Autodesk Inventor part; units mm, degrees
(part 5 of 15)
  line L847 (11.116, -14.792) -> (11.116, -15.808)
  arc A1970 (11.0652, -15.808) -> (11.1668, -15.808) centre (11.116, -15.808) ccw
  arc A1971 (11.1668, -14.792) -> (11.0652, -14.792) centre (11.116, -14.792) ccw
  arc A1972 (66.7332, 38.092) -> (66.8348, 38.092) centre (66.784, 38.092) ccw
  line L848 (7.084, -14.792) -> (9.116, -14.792)
  arc A1973 (9.116, -14.8428) -> (9.116, -14.7412) centre (9.116, -14.792) ccw
  arc A1974 (7.084, -14.7412) -> (7.084, -14.8428) centre (7.084, -14.792) ccw
  line L849 (9.116, -14.792) -> (9.116, -15.808)
  arc A1975 (9.0652, -15.808) -> (9.1668, -15.808) centre (9.116, -15.808) ccw
  arc A1976 (9.1668, -14.792) -> (9.0652, -14.792) centre (9.116, -14.792) ccw
  line L850 (9.116, -15.808) -> (7.084, -15.808)
  arc A1977 (7.084, -15.7572) -> (7.084, -15.8588) centre (7.084, -15.808) ccw
  arc A1978 (9.116, -15.8588) -> (9.116, -15.7572) centre (9.116, -15.808) ccw
  line L851 (7.084, -15.808) -> (7.084, -14.792)
  arc A1979 (7.1348, -14.792) -> (7.0332, -14.792) centre (7.084, -14.792) ccw
  arc A1980 (7.0332, -15.808) -> (7.1348, -15.808) centre (7.084, -15.808) ccw
  line L852 (5.316, 47.992) -> (3.284, 47.992)
  line L853 (11.116, -23.808) -> (9.084, -23.808)
  arc A1981 (9.084, -23.7572) -> (9.084, -23.8588) centre (9.084, -23.808) ccw
  arc A1982 (11.116, -23.8588) -> (11.116, -23.7572) centre (11.116, -23.808) ccw
  line L854 (9.084, -23.808) -> (9.084, -22.792)
  arc A1983 (9.1348, -22.792) -> (9.0332, -22.792) centre (9.084, -22.792) ccw
  arc A1984 (9.0332, -23.808) -> (9.1348, -23.808) centre (9.084, -23.808) ccw
  line L855 (9.084, -22.792) -> (11.116, -22.792)
  arc A1985 (11.116, -22.8428) -> (11.116, -22.7412) centre (11.116, -22.792) ccw
  arc A1986 (9.084, -22.7412) -> (9.084, -22.8428) centre (9.084, -22.792) ccw
  line L856 (11.116, -22.792) -> (11.116, -23.808)
  arc A1987 (11.0652, -23.808) -> (11.1668, -23.808) centre (11.116, -23.808) ccw
  arc A1988 (11.1668, -22.792) -> (11.0652, -22.792) centre (11.116, -22.792) ccw
  arc A1989 (3.284, 48.0428) -> (3.284, 47.9412) centre (3.284, 47.992) ccw
  line L857 (9.116, -23.808) -> (7.084, -23.808)
  arc A1990 (7.084, -23.7572) -> (7.084, -23.8588) centre (7.084, -23.808) ccw
  arc A1991 (9.116, -23.8588) -> (9.116, -23.7572) centre (9.116, -23.808) ccw
  line L858 (7.084, -23.808) -> (7.084, -22.792)
  arc A1992 (7.1348, -22.792) -> (7.0332, -22.792) centre (7.084, -22.792) ccw
  arc A1993 (7.0332, -23.808) -> (7.1348, -23.808) centre (7.084, -23.808) ccw
  line L859 (7.084, -22.792) -> (9.116, -22.792)
  arc A1994 (9.116, -22.8428) -> (9.116, -22.7412) centre (9.116, -22.792) ccw
  arc A1995 (7.084, -22.7412) -> (7.084, -22.8428) centre (7.084, -22.792) ccw
  line L860 (9.116, -22.792) -> (9.116, -23.808)
  arc A1996 (9.0652, -23.808) -> (9.1668, -23.808) centre (9.116, -23.808) ccw
  arc A1997 (9.1668, -22.792) -> (9.0652, -22.792) centre (9.116, -22.792) ccw
  arc A1998 (5.316, 47.9412) -> (5.316, 48.0428) centre (5.316, 47.992) ccw
  line L861 (8.884, -18.292) -> (10.916, -18.292)
  arc A1999 (10.916, -18.3428) -> (10.916, -18.2412) centre (10.916, -18.292) ccw
  arc A2000 (8.884, -18.2412) -> (8.884, -18.3428) centre (8.884, -18.292) ccw
  line L862 (10.916, -18.292) -> (10.916, -19.308)
  arc A2001 (10.8652, -19.308) -> (10.9668, -19.308) centre (10.916, -19.308) ccw
  arc A2002 (10.9668, -18.292) -> (10.8652, -18.292) centre (10.916, -18.292) ccw
  line L863 (10.916, -19.308) -> (8.884, -19.308)
  arc A2003 (8.884, -19.2572) -> (8.884, -19.3588) centre (8.884, -19.308) ccw
  arc A2004 (10.916, -19.3588) -> (10.916, -19.2572) centre (10.916, -19.308) ccw
  line L864 (8.884, -19.308) -> (8.884, -18.292)
  arc A2005 (8.9348, -18.292) -> (8.8332, -18.292) centre (8.884, -18.292) ccw
  arc A2006 (8.8332, -19.308) -> (8.9348, -19.308) centre (8.884, -19.308) ccw
  line L865 (3.284, 47.992) -> (3.284, 49.008)
  line L866 (0.916, -15.808) -> (-1.116, -15.808)
  arc A2007 (-1.116, -15.7572) -> (-1.116, -15.8588) centre (-1.116, -15.808) ccw
  arc A2008 (0.916, -15.8588) -> (0.916, -15.7572) centre (0.916, -15.808) ccw
  line L867 (-1.116, -15.808) -> (-1.116, -14.792)
  arc A2009 (-1.0652, -14.792) -> (-1.1668, -14.792) centre (-1.116, -14.792) ccw
  arc A2010 (-1.1668, -15.808) -> (-1.0652, -15.808) centre (-1.116, -15.808) ccw
  line L868 (-1.116, -14.792) -> (0.916, -14.792)
  arc A2011 (0.916, -14.8428) -> (0.916, -14.7412) centre (0.916, -14.792) ccw
  arc A2012 (-1.116, -14.7412) -> (-1.116, -14.8428) centre (-1.116, -14.792) ccw
  line L869 (0.916, -14.792) -> (0.916, -15.808)
  arc A2013 (0.8652, -15.808) -> (0.9668, -15.808) centre (0.916, -15.808) ccw
  arc A2014 (0.9668, -14.792) -> (0.8652, -14.792) centre (0.916, -14.792) ccw
  arc A2015 (3.3348, 49.008) -> (3.2332, 49.008) centre (3.284, 49.008) ccw
  line L870 (4.916, -15.808) -> (2.884, -15.808)
  arc A2016 (2.884, -15.7572) -> (2.884, -15.8588) centre (2.884, -15.808) ccw
  arc A2017 (4.916, -15.8588) -> (4.916, -15.7572) centre (4.916, -15.808) ccw
  line L871 (2.884, -15.808) -> (2.884, -14.792)
  arc A2018 (2.9348, -14.792) -> (2.8332, -14.792) centre (2.884, -14.792) ccw
  arc A2019 (2.8332, -15.808) -> (2.9348, -15.808) centre (2.884, -15.808) ccw
  line L872 (2.884, -14.792) -> (4.916, -14.792)
  arc A2020 (4.916, -14.8428) -> (4.916, -14.7412) centre (4.916, -14.792) ccw
  arc A2021 (2.884, -14.7412) -> (2.884, -14.8428) centre (2.884, -14.792) ccw
  line L873 (4.916, -14.792) -> (4.916, -15.808)
  arc A2022 (4.8652, -15.808) -> (4.9668, -15.808) centre (4.916, -15.808) ccw
  arc A2023 (4.9668, -14.792) -> (4.8652, -14.792) centre (4.916, -14.792) ccw
  arc A2024 (3.2332, 47.992) -> (3.3348, 47.992) centre (3.284, 47.992) ccw
  line L874 (8.884, -19.292) -> (10.916, -19.292)
  arc A2025 (10.916, -19.3428) -> (10.916, -19.2412) centre (10.916, -19.292) ccw
  arc A2026 (8.884, -19.2412) -> (8.884, -19.3428) centre (8.884, -19.292) ccw
  line L875 (10.916, -19.292) -> (10.916, -20.308)
  arc A2027 (10.8652, -20.308) -> (10.9668, -20.308) centre (10.916, -20.308) ccw
  arc A2028 (10.9668, -19.292) -> (10.8652, -19.292) centre (10.916, -19.292) ccw
  line L876 (10.916, -20.308) -> (8.884, -20.308)
  arc A2029 (8.884, -20.2572) -> (8.884, -20.3588) centre (8.884, -20.308) ccw
  arc A2030 (10.916, -20.3588) -> (10.916, -20.2572) centre (10.916, -20.308) ccw
  line L877 (8.884, -20.308) -> (8.884, -19.292)
  arc A2031 (8.9348, -19.292) -> (8.8332, -19.292) centre (8.884, -19.292) ccw
  arc A2032 (8.8332, -20.308) -> (8.9348, -20.308) centre (8.884, -20.308) ccw
  line L878 (3.284, 49.008) -> (5.316, 49.008)
  line L879 (2.916, -23.808) -> (0.884, -23.808)
  arc A2033 (0.884, -23.7572) -> (0.884, -23.8588) centre (0.884, -23.808) ccw
  arc A2034 (2.916, -23.8588) -> (2.916, -23.7572) centre (2.916, -23.808) ccw
  line L880 (0.884, -23.808) -> (0.884, -22.792)
  arc A2035 (0.9348, -22.792) -> (0.8332, -22.792) centre (0.884, -22.792) ccw
  arc A2036 (0.8332, -23.808) -> (0.9348, -23.808) centre (0.884, -23.808) ccw
  line L881 (0.884, -22.792) -> (2.916, -22.792)
  arc A2037 (2.916, -22.8428) -> (2.916, -22.7412) centre (2.916, -22.792) ccw
  arc A2038 (0.884, -22.7412) -> (0.884, -22.8428) centre (0.884, -22.792) ccw
  line L882 (2.916, -22.792) -> (2.916, -23.808)
  arc A2039 (2.8652, -23.808) -> (2.9668, -23.808) centre (2.916, -23.808) ccw
  arc A2040 (2.9668, -22.792) -> (2.8652, -22.792) centre (2.916, -22.792) ccw
  arc A2041 (5.316, 48.9572) -> (5.316, 49.0588) centre (5.316, 49.008) ccw
  line L883 (0.916, -23.808) -> (-1.116, -23.808)
  arc A2042 (-1.116, -23.7572) -> (-1.116, -23.8588) centre (-1.116, -23.808) ccw
  arc A2043 (0.916, -23.8588) -> (0.916, -23.7572) centre (0.916, -23.808) ccw
  line L884 (-1.116, -23.808) -> (-1.116, -22.792)
  arc A2044 (-1.0652, -22.792) -> (-1.1668, -22.792) centre (-1.116, -22.792) ccw
  arc A2045 (-1.1668, -23.808) -> (-1.0652, -23.808) centre (-1.116, -23.808) ccw
  line L885 (-1.116, -22.792) -> (0.916, -22.792)
  arc A2046 (0.916, -22.8428) -> (0.916, -22.7412) centre (0.916, -22.792) ccw
  arc A2047 (-1.116, -22.7412) -> (-1.116, -22.8428) centre (-1.116, -22.792) ccw
  line L886 (0.916, -22.792) -> (0.916, -23.808)
  arc A2048 (0.8652, -23.808) -> (0.9668, -23.808) centre (0.916, -23.808) ccw
  arc A2049 (0.9668, -22.792) -> (0.8652, -22.792) centre (0.916, -22.792) ccw
  arc A2050 (3.284, 49.0588) -> (3.284, 48.9572) centre (3.284, 49.008) ccw
  line L887 (3.716, -19.808) -> (1.684, -19.808)
  arc A2051 (1.684, -19.7572) -> (1.684, -19.8588) centre (1.684, -19.808) ccw
  arc A2052 (3.716, -19.8588) -> (3.716, -19.7572) centre (3.716, -19.808) ccw
  line L888 (1.684, -19.808) -> (1.684, -18.792)
  arc A2053 (1.7348, -18.792) -> (1.6332, -18.792) centre (1.684, -18.792) ccw
  arc A2054 (1.6332, -19.808) -> (1.7348, -19.808) centre (1.684, -19.808) ccw
  line L889 (1.684, -18.792) -> (3.716, -18.792)
  arc A2055 (3.716, -18.8428) -> (3.716, -18.7412) centre (3.716, -18.792) ccw
  arc A2056 (1.684, -18.7412) -> (1.684, -18.8428) centre (1.684, -18.792) ccw
  line L890 (3.716, -18.792) -> (3.716, -19.808)
  arc A2057 (3.6652, -19.808) -> (3.7668, -19.808) centre (3.716, -19.808) ccw
  arc A2058 (3.7668, -18.792) -> (3.6652, -18.792) centre (3.716, -18.792) ccw
  line L891 (5.316, 49.008) -> (5.316, 47.992)
  line L892 (-11.108, -24.116) -> (-11.108, -22.084)
  arc A2059 (-11.0572, -22.084) -> (-11.1588, -22.084) centre (-11.108, -22.084) ccw
  arc A2060 (-11.1588, -24.116) -> (-11.0572, -24.116) centre (-11.108, -24.116) ccw
  line L893 (-11.108, -22.084) -> (-10.092, -22.084)
  arc A2061 (-10.092, -22.1348) -> (-10.092, -22.0332) centre (-10.092, -22.084) ccw
  arc A2062 (-11.108, -22.0332) -> (-11.108, -22.1348) centre (-11.108, -22.084) ccw
  line L894 (-10.092, -22.084) -> (-10.092, -24.116)
  arc A2063 (-10.1428, -24.116) -> (-10.0412, -24.116) centre (-10.092, -24.116) ccw
  arc A2064 (-10.0412, -22.084) -> (-10.1428, -22.084) centre (-10.092, -22.084) ccw
  line L895 (-10.092, -24.116) -> (-11.108, -24.116)
  arc A2065 (-11.108, -24.0652) -> (-11.108, -24.1668) centre (-11.108, -24.116) ccw
  arc A2066 (-10.092, -24.1668) -> (-10.092, -24.0652) centre (-10.092, -24.116) ccw
  arc A2067 (5.2652, 47.992) -> (5.3668, 47.992) centre (5.316, 47.992) ccw
  line L896 (-22.292, 42.016) -> (-22.292, 39.984)
  arc A2068 (-22.3428, 39.984) -> (-22.2412, 39.984) centre (-22.292, 39.984) ccw
  arc A2069 (-22.2412, 42.016) -> (-22.3428, 42.016) centre (-22.292, 42.016) ccw
  line L897 (-22.292, 39.984) -> (-23.308, 39.984)
  arc A2070 (-23.308, 40.0348) -> (-23.308, 39.9332) centre (-23.308, 39.984) ccw
  arc A2071 (-22.292, 39.9332) -> (-22.292, 40.0348) centre (-22.292, 39.984) ccw
  line L898 (-23.308, 39.984) -> (-23.308, 42.016)
  arc A2072 (-23.2572, 42.016) -> (-23.3588, 42.016) centre (-23.308, 42.016) ccw
  arc A2073 (-23.3588, 39.984) -> (-23.2572, 39.984) centre (-23.308, 39.984) ccw
  line L899 (-23.308, 42.016) -> (-22.292, 42.016)
  arc A2074 (-22.292, 41.9652) -> (-22.292, 42.0668) centre (-22.292, 42.016) ccw
  arc A2075 (-23.308, 42.0668) -> (-23.308, 41.9652) centre (-23.308, 42.016) ccw
  arc A2076 (5.3668, 49.008) -> (5.2652, 49.008) centre (5.316, 49.008) ccw
  line L900 (-18.092, 44.016) -> (-18.092, 41.984)
  arc A2077 (-18.1428, 41.984) -> (-18.0412, 41.984) centre (-18.092, 41.984) ccw
  arc A2078 (-18.0412, 44.016) -> (-18.1428, 44.016) centre (-18.092, 44.016) ccw
  line L901 (-18.092, 41.984) -> (-19.108, 41.984)
  arc A2079 (-19.108, 42.0348) -> (-19.108, 41.9332) centre (-19.108, 41.984) ccw
  arc A2080 (-18.092, 41.9332) -> (-18.092, 42.0348) centre (-18.092, 41.984) ccw
  line L902 (-19.108, 41.984) -> (-19.108, 44.016)
  arc A2081 (-19.0572, 44.016) -> (-19.1588, 44.016) centre (-19.108, 44.016) ccw
  arc A2082 (-19.1588, 41.984) -> (-19.0572, 41.984) centre (-19.108, 41.984) ccw
  line L903 (-19.108, 44.016) -> (-18.092, 44.016)
  arc A2083 (-18.092, 43.9652) -> (-18.092, 44.0668) centre (-18.092, 44.016) ccw
  arc A2084 (-19.108, 44.0668) -> (-19.108, 43.9652) centre (-19.108, 44.016) ccw
  line L904 (5.584, 49.008) -> (7.616, 49.008)
  line L905 (-21.284, 38.992) -> (-23.316, 38.992)
  arc A2085 (-23.316, 39.0428) -> (-23.316, 38.9412) centre (-23.316, 38.992) ccw
  arc A2086 (-21.284, 38.9412) -> (-21.284, 39.0428) centre (-21.284, 38.992) ccw
  line L906 (-23.316, 38.992) -> (-23.316, 40.008)
  arc A2087 (-23.2652, 40.008) -> (-23.3668, 40.008) centre (-23.316, 40.008) ccw
  arc A2088 (-23.3668, 38.992) -> (-23.2652, 38.992) centre (-23.316, 38.992) ccw
  line L907 (-23.316, 40.008) -> (-21.284, 40.008)
  arc A2089 (-21.284, 39.9572) -> (-21.284, 40.0588) centre (-21.284, 40.008) ccw
  arc A2090 (-23.316, 40.0588) -> (-23.316, 39.9572) centre (-23.316, 40.008) ccw
  line L908 (-21.284, 40.008) -> (-21.284, 38.992)
  arc A2091 (-21.3348, 38.992) -> (-21.2332, 38.992) centre (-21.284, 38.992) ccw
  arc A2092 (-21.2332, 40.008) -> (-21.3348, 40.008) centre (-21.284, 40.008) ccw
  arc A2093 (7.616, 48.9572) -> (7.616, 49.0588) centre (7.616, 49.008) ccw
  line L909 (-22.016, 50.108) -> (-19.984, 50.108)
  arc A2094 (-19.984, 50.0572) -> (-19.984, 50.1588) centre (-19.984, 50.108) ccw
  arc A2095 (-22.016, 50.1588) -> (-22.016, 50.0572) centre (-22.016, 50.108) ccw
  line L910 (-19.984, 50.108) -> (-19.984, 49.092)
  arc A2096 (-20.0348, 49.092) -> (-19.9332, 49.092) centre (-19.984, 49.092) ccw
  arc A2097 (-19.9332, 50.108) -> (-20.0348, 50.108) centre (-19.984, 50.108) ccw
  line L911 (-19.984, 49.092) -> (-22.016, 49.092)
  arc A2098 (-22.016, 49.1428) -> (-22.016, 49.0412) centre (-22.016, 49.092) ccw
  arc A2099 (-19.984, 49.0412) -> (-19.984, 49.1428) centre (-19.984, 49.092) ccw
  line L912 (-22.016, 49.092) -> (-22.016, 50.108)
  arc A2100 (-21.9652, 50.108) -> (-22.0668, 50.108) centre (-22.016, 50.108) ccw
  arc A2101 (-22.0668, 49.092) -> (-21.9652, 49.092) centre (-22.016, 49.092) ccw
  arc A2102 (5.584, 49.0588) -> (5.584, 48.9572) centre (5.584, 49.008) ccw
  line L913 (-19.916, 41.508) -> (-17.884, 41.508)
  arc A2103 (-17.884, 41.4572) -> (-17.884, 41.5588) centre (-17.884, 41.508) ccw
  arc A2104 (-19.916, 41.5588) -> (-19.916, 41.4572) centre (-19.916, 41.508) ccw
  line L914 (-17.884, 41.508) -> (-17.884, 40.492)
  arc A2105 (-17.9348, 40.492) -> (-17.8332, 40.492) centre (-17.884, 40.492) ccw
  arc A2106 (-17.8332, 41.508) -> (-17.9348, 41.508) centre (-17.884, 41.508) ccw
  line L915 (-17.884, 40.492) -> (-19.916, 40.492)
  arc A2107 (-19.916, 40.5428) -> (-19.916, 40.4412) centre (-19.916, 40.492) ccw
  arc A2108 (-17.884, 40.4412) -> (-17.884, 40.5428) centre (-17.884, 40.492) ccw
  line L916 (-19.916, 40.492) -> (-19.916, 41.508)
  arc A2109 (-19.8652, 41.508) -> (-19.9668, 41.508) centre (-19.916, 41.508) ccw
  arc A2110 (-19.9668, 40.492) -> (-19.8652, 40.492) centre (-19.916, 40.492) ccw
  line L917 (7.616, 49.008) -> (7.616, 47.992)
  line L918 (-22.292, 44.016) -> (-22.292, 41.984)
  arc A2111 (-22.3428, 41.984) -> (-22.2412, 41.984) centre (-22.292, 41.984) ccw
  arc A2112 (-22.2412, 44.016) -> (-22.3428, 44.016) centre (-22.292, 44.016) ccw
  line L919 (-22.292, 41.984) -> (-23.308, 41.984)
  arc A2113 (-23.308, 42.0348) -> (-23.308, 41.9332) centre (-23.308, 41.984) ccw
  arc A2114 (-22.292, 41.9332) -> (-22.292, 42.0348) centre (-22.292, 41.984) ccw
  line L920 (-23.308, 41.984) -> (-23.308, 44.016)
  arc A2115 (-23.2572, 44.016) -> (-23.3588, 44.016) centre (-23.308, 44.016) ccw
  arc A2116 (-23.3588, 41.984) -> (-23.2572, 41.984) centre (-23.308, 41.984) ccw
  line L921 (-23.308, 44.016) -> (-22.292, 44.016)
  arc A2117 (-22.292, 43.9652) -> (-22.292, 44.0668) centre (-22.292, 44.016) ccw
  arc A2118 (-23.308, 44.0668) -> (-23.308, 43.9652) centre (-23.308, 44.016) ccw
  arc A2119 (7.5652, 47.992) -> (7.6668, 47.992) centre (7.616, 47.992) ccw
  line L922 (-20.292, 44.016) -> (-20.292, 41.984)
  arc A2120 (-20.3428, 41.984) -> (-20.2412, 41.984) centre (-20.292, 41.984) ccw
  arc A2121 (-20.2412, 44.016) -> (-20.3428, 44.016) centre (-20.292, 44.016) ccw
  line L923 (-20.292, 41.984) -> (-21.308, 41.984)
  arc A2122 (-21.308, 42.0348) -> (-21.308, 41.9332) centre (-21.308, 41.984) ccw
  arc A2123 (-20.292, 41.9332) -> (-20.292, 42.0348) centre (-20.292, 41.984) ccw
  line L924 (-21.308, 41.984) -> (-21.308, 44.016)
  arc A2124 (-21.2572, 44.016) -> (-21.3588, 44.016) centre (-21.308, 44.016) ccw
  arc A2125 (-21.3588, 41.984) -> (-21.2572, 41.984) centre (-21.308, 41.984) ccw
  line L925 (-21.308, 44.016) -> (-20.292, 44.016)
  arc A2126 (-20.292, 43.9652) -> (-20.292, 44.0668) centre (-20.292, 44.016) ccw
  arc A2127 (-21.308, 44.0668) -> (-21.308, 43.9652) centre (-21.308, 44.016) ccw
  arc A2128 (7.6668, 49.008) -> (7.5652, 49.008) centre (7.616, 49.008) ccw
  line L926 (-21.292, 44.016) -> (-21.292, 41.984)
  arc A2129 (-21.3428, 41.984) -> (-21.2412, 41.984) centre (-21.292, 41.984) ccw
  arc A2130 (-21.2412, 44.016) -> (-21.3428, 44.016) centre (-21.292, 44.016) ccw
  line L927 (-21.292, 41.984) -> (-22.308, 41.984)
  arc A2131 (-22.308, 42.0348) -> (-22.308, 41.9332) centre (-22.308, 41.984) ccw
  arc A2132 (-21.292, 41.9332) -> (-21.292, 42.0348) centre (-21.292, 41.984) ccw
  line L928 (-22.308, 41.984) -> (-22.308, 44.016)
  arc A2133 (-22.2572, 44.016) -> (-22.3588, 44.016) centre (-22.308, 44.016) ccw
  arc A2134 (-22.3588, 41.984) -> (-22.2572, 41.984) centre (-22.308, 41.984) ccw
  line L929 (-22.308, 44.016) -> (-21.292, 44.016)
  arc A2135 (-21.292, 43.9652) -> (-21.292, 44.0668) centre (-21.292, 44.016) ccw
  arc A2136 (-22.308, 44.0668) -> (-22.308, 43.9652) centre (-22.308, 44.016) ccw
  line L930 (7.616, 47.992) -> (5.584, 47.992)
  line L931 (-17.897, 40.935) -> (-15.103, 40.935)
  arc A2137 (-15.103, 40.8842) -> (-15.103, 40.9858) centre (-15.103, 40.935) ccw
  arc A2138 (-17.897, 40.9858) -> (-17.897, 40.8842) centre (-17.897, 40.935) ccw
  line L932 (-15.103, 40.935) -> (-15.103, 39.665)
  arc A2139 (-15.1538, 39.665) -> (-15.0522, 39.665) centre (-15.103, 39.665) ccw
  arc A2140 (-15.0522, 40.935) -> (-15.1538, 40.935) centre (-15.103, 40.935) ccw
  line L933 (-15.103, 39.665) -> (-17.897, 39.665)
  arc A2141 (-17.897, 39.7158) -> (-17.897, 39.6142) centre (-17.897, 39.665) ccw
  arc A2142 (-15.103, 39.6142) -> (-15.103, 39.7158) centre (-15.103, 39.665) ccw
  line L934 (-17.897, 39.665) -> (-17.897, 40.935)
  arc A2143 (-17.8462, 40.935) -> (-17.9478, 40.935) centre (-17.897, 40.935) ccw
  arc A2144 (-17.9478, 39.665) -> (-17.8462, 39.665) centre (-17.897, 39.665) ccw
  arc A2145 (5.584, 48.0428) -> (5.584, 47.9412) centre (5.584, 47.992) ccw
  line L935 (-17.516, 42.008) -> (-15.484, 42.008)
  arc A2146 (-15.484, 41.9572) -> (-15.484, 42.0588) centre (-15.484, 42.008) ccw
  arc A2147 (-17.516, 42.0588) -> (-17.516, 41.9572) centre (-17.516, 42.008) ccw
  line L936 (-15.484, 42.008) -> (-15.484, 40.992)
  arc A2148 (-15.5348, 40.992) -> (-15.4332, 40.992) centre (-15.484, 40.992) ccw
  arc A2149 (-15.4332, 42.008) -> (-15.5348, 42.008) centre (-15.484, 42.008) ccw
  line L937 (-15.484, 40.992) -> (-17.516, 40.992)
  arc A2150 (-17.516, 41.0428) -> (-17.516, 40.9412) centre (-17.516, 40.992) ccw
  arc A2151 (-15.484, 40.9412) -> (-15.484, 41.0428) centre (-15.484, 40.992) ccw
  line L938 (-17.516, 40.992) -> (-17.516, 42.008)
  arc A2152 (-17.4652, 42.008) -> (-17.5668, 42.008) centre (-17.516, 42.008) ccw
  arc A2153 (-17.5668, 40.992) -> (-17.4652, 40.992) centre (-17.516, 40.992) ccw
  arc A2154 (7.616, 47.9412) -> (7.616, 48.0428) centre (7.616, 47.992) ccw
  line L939 (2.616, -52.308) -> (0.584, -52.308)
  arc A2155 (0.584, -52.2572) -> (0.584, -52.3588) centre (0.584, -52.308) ccw
  arc A2156 (2.616, -52.3588) -> (2.616, -52.2572) centre (2.616, -52.308) ccw
  line L940 (0.584, -52.308) -> (0.584, -51.292)
  arc A2157 (0.6348, -51.292) -> (0.5332, -51.292) centre (0.584, -51.292) ccw
  arc A2158 (0.5332, -52.308) -> (0.6348, -52.308) centre (0.584, -52.308) ccw
  line L941 (0.584, -51.292) -> (2.616, -51.292)
  arc A2159 (2.616, -51.3428) -> (2.616, -51.2412) centre (2.616, -51.292) ccw
  arc A2160 (0.584, -51.2412) -> (0.584, -51.3428) centre (0.584, -51.292) ccw
  line L942 (2.616, -51.292) -> (2.616, -52.308)
  arc A2161 (2.5652, -52.308) -> (2.6668, -52.308) centre (2.616, -52.308) ccw
  arc A2162 (2.6668, -51.292) -> (2.5652, -51.292) centre (2.616, -51.292) ccw
  line L943 (5.584, 47.992) -> (5.584, 49.008)
  line L944 (7.892, -53.216) -> (7.892, -51.184)
  arc A2163 (7.9428, -51.184) -> (7.8412, -51.184) centre (7.892, -51.184) ccw
  arc A2164 (7.8412, -53.216) -> (7.9428, -53.216) centre (7.892, -53.216) ccw
  line L945 (7.892, -51.184) -> (8.908, -51.184)
  arc A2165 (8.908, -51.2348) -> (8.908, -51.1332) centre (8.908, -51.184) ccw
  arc A2166 (7.892, -51.1332) -> (7.892, -51.2348) centre (7.892, -51.184) ccw
  line L946 (8.908, -51.184) -> (8.908, -53.216)
  arc A2167 (8.8572, -53.216) -> (8.9588, -53.216) centre (8.908, -53.216) ccw
  arc A2168 (8.9588, -51.184) -> (8.8572, -51.184) centre (8.908, -51.184) ccw
  line L947 (8.908, -53.216) -> (7.892, -53.216)
  arc A2169 (7.892, -53.1652) -> (7.892, -53.2668) centre (7.892, -53.216) ccw
  arc A2170 (8.908, -53.2668) -> (8.908, -53.1652) centre (8.908, -53.216) ccw
  arc A2171 (5.6348, 49.008) -> (5.5332, 49.008) centre (5.584, 49.008) ccw
  line L948 (2.584, -48.292) -> (4.616, -48.292)
  arc A2172 (4.616, -48.3428) -> (4.616, -48.2412) centre (4.616, -48.292) ccw
  arc A2173 (2.584, -48.2412) -> (2.584, -48.3428) centre (2.584, -48.292) ccw
  line L949 (4.616, -48.292) -> (4.616, -49.308)
  arc A2174 (4.5652, -49.308) -> (4.6668, -49.308) centre (4.616, -49.308) ccw
  arc A2175 (4.6668, -48.292) -> (4.5652, -48.292) centre (4.616, -48.292) ccw
  line L950 (4.616, -49.308) -> (2.584, -49.308)
  arc A2176 (2.584, -49.2572) -> (2.584, -49.3588) centre (2.584, -49.308) ccw
  arc A2177 (4.616, -49.3588) -> (4.616, -49.2572) centre (4.616, -49.308) ccw
  line L951 (2.584, -49.308) -> (2.584, -48.292)
  arc A2178 (2.6348, -48.292) -> (2.5332, -48.292) centre (2.584, -48.292) ccw
  arc A2179 (2.5332, -49.308) -> (2.6348, -49.308) centre (2.584, -49.308) ccw
  arc A2180 (5.5332, 47.992) -> (5.6348, 47.992) centre (5.584, 47.992) ccw
  line L952 (2.616, -50.308) -> (0.584, -50.308)
  arc A2181 (0.584, -50.2572) -> (0.584, -50.3588) centre (0.584, -50.308) ccw
  arc A2182 (2.616, -50.3588) -> (2.616, -50.2572) centre (2.616, -50.308) ccw
  line L953 (0.584, -50.308) -> (0.584, -49.292)
  arc A2183 (0.6348, -49.292) -> (0.5332, -49.292) centre (0.584, -49.292) ccw
  arc A2184 (0.5332, -50.308) -> (0.6348, -50.308) centre (0.584, -50.308) ccw
  line L954 (0.584, -49.292) -> (2.616, -49.292)
  arc A2185 (2.616, -49.3428) -> (2.616, -49.2412) centre (2.616, -49.292) ccw
  arc A2186 (0.584, -49.2412) -> (0.584, -49.3428) centre (0.584, -49.292) ccw
  line L955 (2.616, -49.292) -> (2.616, -50.308)
  arc A2187 (2.5652, -50.308) -> (2.6668, -50.308) centre (2.616, -50.308) ccw
  arc A2188 (2.6668, -49.292) -> (2.5652, -49.292) centre (2.616, -49.292) ccw
  line L956 (-3.245, -53.28) -> (-18.355, -53.28)
  line L957 (10.284, -47.792) -> (12.316, -47.792)
  arc A2189 (12.316, -47.8428) -> (12.316, -47.7412) centre (12.316, -47.792) ccw
  arc A2190 (10.284, -47.7412) -> (10.284, -47.8428) centre (10.284, -47.792) ccw
  line L958 (12.316, -47.792) -> (12.316, -48.808)
  arc A2191 (12.2652, -48.808) -> (12.3668, -48.808) centre (12.316, -48.808) ccw
  arc A2192 (12.3668, -47.792) -> (12.2652, -47.792) centre (12.316, -47.792) ccw
  line L959 (12.316, -48.808) -> (10.284, -48.808)
  arc A2193 (10.284, -48.7572) -> (10.284, -48.8588) centre (10.284, -48.808) ccw
  arc A2194 (12.316, -48.8588) -> (12.316, -48.7572) centre (12.316, -48.808) ccw
  line L960 (10.284, -48.808) -> (10.284, -47.792)
  arc A2195 (10.3348, -47.792) -> (10.2332, -47.792) centre (10.284, -47.792) ccw
  arc A2196 (10.2332, -48.808) -> (10.3348, -48.808) centre (10.284, -48.808) ccw
  arc A2197 (-18.355, -53.2482) -> (-18.355, -53.3117) centre (-18.355, -53.28) ccw
  line L961 (10.116, -50.808) -> (8.084, -50.808)
  arc A2198 (8.084, -50.7572) -> (8.084, -50.8588) centre (8.084, -50.808) ccw
  arc A2199 (10.116, -50.8588) -> (10.116, -50.7572) centre (10.116, -50.808) ccw
  line L962 (8.084, -50.808) -> (8.084, -49.792)
  arc A2200 (8.1348, -49.792) -> (8.0332, -49.792) centre (8.084, -49.792) ccw
  arc A2201 (8.0332, -50.808) -> (8.1348, -50.808) centre (8.084, -50.808) ccw
  line L963 (8.084, -49.792) -> (10.116, -49.792)
  arc A2202 (10.116, -49.8428) -> (10.116, -49.7412) centre (10.116, -49.792) ccw
  arc A2203 (8.084, -49.7412) -> (8.084, -49.8428) centre (8.084, -49.792) ccw
  line L964 (10.116, -49.792) -> (10.116, -50.808)
  arc A2204 (10.0652, -50.808) -> (10.1668, -50.808) centre (10.116, -50.808) ccw
  arc A2205 (10.1668, -49.792) -> (10.0652, -49.792) centre (10.116, -49.792) ccw
  arc A2206 (-3.245, -53.3117) -> (-3.245, -53.2482) centre (-3.245, -53.28) ccw
  line L965 (2.616, -49.308) -> (0.584, -49.308)
  arc A2207 (0.584, -49.2572) -> (0.584, -49.3588) centre (0.584, -49.308) ccw
  arc A2208 (2.616, -49.3588) -> (2.616, -49.2572) centre (2.616, -49.308) ccw
  line L966 (0.584, -49.308) -> (0.584, -48.292)
  arc A2209 (0.6348, -48.292) -> (0.5332, -48.292) centre (0.584, -48.292) ccw
  arc A2210 (0.5332, -49.308) -> (0.6348, -49.308) centre (0.584, -49.308) ccw
  line L967 (0.584, -48.292) -> (2.616, -48.292)
  arc A2211 (2.616, -48.3428) -> (2.616, -48.2412) centre (2.616, -48.292) ccw
  arc A2212 (0.584, -48.2412) -> (0.584, -48.3428) centre (0.584, -48.292) ccw
  line L968 (2.616, -48.292) -> (2.616, -49.308)
  arc A2213 (2.5652, -49.308) -> (2.6668, -49.308) centre (2.616, -49.308) ccw
  arc A2214 (2.6668, -48.292) -> (2.5652, -48.292) centre (2.616, -48.292) ccw
  line L969 (-18.355, -40.12) -> (-3.245, -40.12)
  line L970 (7.608, -45.784) -> (7.608, -47.816)
  arc A2215 (7.5572, -47.816) -> (7.6588, -47.816) centre (7.608, -47.816) ccw
  arc A2216 (7.6588, -45.784) -> (7.5572, -45.784) centre (7.608, -45.784) ccw
  line L971 (7.608, -47.816) -> (6.592, -47.816)
  arc A2217 (6.592, -47.7652) -> (6.592, -47.8668) centre (6.592, -47.816) ccw
  arc A2218 (7.608, -47.8668) -> (7.608, -47.7652) centre (7.608, -47.816) ccw
  line L972 (6.592, -47.816) -> (6.592, -45.784)
  arc A2219 (6.6428, -45.784) -> (6.5412, -45.784) centre (6.592, -45.784) ccw
  arc A2220 (6.5412, -47.816) -> (6.6428, -47.816) centre (6.592, -47.816) ccw
  line L973 (6.592, -45.784) -> (7.608, -45.784)
  arc A2221 (7.608, -45.8348) -> (7.608, -45.7332) centre (7.608, -45.784) ccw
  arc A2222 (6.592, -45.7332) -> (6.592, -45.8348) centre (6.592, -45.784) ccw
  arc A2223 (-3.245, -40.1517) -> (-3.245, -40.0882) centre (-3.245, -40.12) ccw
  line L974 (5.892, -53.216) -> (5.892, -51.184)
  arc A2224 (5.9428, -51.184) -> (5.8412, -51.184) centre (5.892, -51.184) ccw
  arc A2225 (5.8412, -53.216) -> (5.9428, -53.216) centre (5.892, -53.216) ccw
  line L975 (5.892, -51.184) -> (6.908, -51.184)
  arc A2226 (6.908, -51.2348) -> (6.908, -51.1332) centre (6.908, -51.184) ccw
  arc A2227 (5.892, -51.1332) -> (5.892, -51.2348) centre (5.892, -51.184) ccw
  line L976 (6.908, -51.184) -> (6.908, -53.216)
  arc A2228 (6.8572, -53.216) -> (6.9588, -53.216) centre (6.908, -53.216) ccw
  arc A2229 (6.9588, -51.184) -> (6.8572, -51.184) centre (6.908, -51.184) ccw
  line L977 (6.908, -53.216) -> (5.892, -53.216)
  arc A2230 (5.892, -53.1652) -> (5.892, -53.2668) centre (5.892, -53.216) ccw
  arc A2231 (6.908, -53.2668) -> (6.908, -53.1652) centre (6.908, -53.216) ccw
  arc A2232 (-18.355, -40.0882) -> (-18.355, -40.1517) centre (-18.355, -40.12) ccw
  line L978 (2.616, -51.308) -> (0.584, -51.308)
  arc A2233 (0.584, -51.2572) -> (0.584, -51.3588) centre (0.584, -51.308) ccw
  arc A2234 (2.616, -51.3588) -> (2.616, -51.2572) centre (2.616, -51.308) ccw
  line L979 (0.584, -51.308) -> (0.584, -50.292)
  arc A2235 (0.6348, -50.292) -> (0.5332, -50.292) centre (0.584, -50.292) ccw
  arc A2236 (0.5332, -51.308) -> (0.6348, -51.308) centre (0.584, -51.308) ccw
  line L980 (0.584, -50.292) -> (2.616, -50.292)
  arc A2237 (2.616, -50.3428) -> (2.616, -50.2412) centre (2.616, -50.292) ccw
  arc A2238 (0.584, -50.2412) -> (0.584, -50.3428) centre (0.584, -50.292) ccw
  line L981 (2.616, -50.292) -> (2.616, -51.308)
  arc A2239 (2.5652, -51.308) -> (2.6668, -51.308) centre (2.616, -51.308) ccw
  arc A2240 (2.6668, -50.292) -> (2.5652, -50.292) centre (2.616, -50.292) ccw
  line L982 (-3.245, -40.12) -> (-3.245, -53.28)
  line L983 (8.892, -53.216) -> (8.892, -51.184)
  arc A2241 (8.9428, -51.184) -> (8.8412, -51.184) centre (8.892, -51.184) ccw
  arc A2242 (8.8412, -53.216) -> (8.9428, -53.216) centre (8.892, -53.216) ccw
  line L984 (8.892, -51.184) -> (9.908, -51.184)
  arc A2243 (9.908, -51.2348) -> (9.908, -51.1332) centre (9.908, -51.184) ccw
  arc A2244 (8.892, -51.1332) -> (8.892, -51.2348) centre (8.892, -51.184) ccw
  line L985 (9.908, -51.184) -> (9.908, -53.216)
  arc A2245 (9.8572, -53.216) -> (9.9588, -53.216) centre (9.908, -53.216) ccw
  arc A2246 (9.9588, -51.184) -> (9.8572, -51.184) centre (9.908, -51.184) ccw
  line L986 (9.908, -53.216) -> (8.892, -53.216)
  arc A2247 (8.892, -53.1652) -> (8.892, -53.2668) centre (8.892, -53.216) ccw
  arc A2248 (9.908, -53.2668) -> (9.908, -53.1652) centre (9.908, -53.216) ccw
  arc A2249 (-3.2767, -53.28) -> (-3.2132, -53.28) centre (-3.245, -53.28) ccw
  line L987 (9.608, -45.784) -> (9.608, -47.816)
  arc A2250 (9.5572, -47.816) -> (9.6588, -47.816) centre (9.608, -47.816) ccw
  arc A2251 (9.6588, -45.784) -> (9.5572, -45.784) centre (9.608, -45.784) ccw
  line L988 (9.608, -47.816) -> (8.592, -47.816)
  arc A2252 (8.592, -47.7652) -> (8.592, -47.8668) centre (8.592, -47.816) ccw
  arc A2253 (9.608, -47.8668) -> (9.608, -47.7652) centre (9.608, -47.816) ccw
  line L989 (8.592, -47.816) -> (8.592, -45.784)
  arc A2254 (8.6428, -45.784) -> (8.5412, -45.784) centre (8.592, -45.784) ccw
  arc A2255 (8.5412, -47.816) -> (8.6428, -47.816) centre (8.592, -47.816) ccw
  line L990 (8.592, -45.784) -> (9.608, -45.784)
  arc A2256 (9.608, -45.8348) -> (9.608, -45.7332) centre (9.608, -45.784) ccw
  arc A2257 (8.592, -45.7332) -> (8.592, -45.8348) centre (8.592, -45.784) ccw
  arc A2258 (-3.2132, -40.12) -> (-3.2767, -40.12) centre (-3.245, -40.12) ccw
  line L991 (4.616, -45.108) -> (2.584, -45.108)
  arc A2259 (2.584, -45.0572) -> (2.584, -45.1588) centre (2.584, -45.108) ccw
  arc A2260 (4.616, -45.1588) -> (4.616, -45.0572) centre (4.616, -45.108) ccw
  line L992 (2.584, -45.108) -> (2.584, -44.092)
  arc A2261 (2.6348, -44.092) -> (2.5332, -44.092) centre (2.584, -44.092) ccw
  arc A2262 (2.5332, -45.108) -> (2.6348, -45.108) centre (2.584, -45.108) ccw
  line L993 (2.584, -44.092) -> (4.616, -44.092)
  arc A2263 (4.616, -44.1428) -> (4.616, -44.0412) centre (4.616, -44.092) ccw
  arc A2264 (2.584, -44.0412) -> (2.584, -44.1428) centre (2.584, -44.092) ccw
  line L994 (4.616, -44.092) -> (4.616, -45.108)
  arc A2265 (4.5652, -45.108) -> (4.6668, -45.108) centre (4.616, -45.108) ccw
  arc A2266 (4.6668, -44.092) -> (4.5652, -44.092) centre (4.616, -44.092) ccw
  line L995 (-18.355, -53.28) -> (-18.355, -40.12)
  line L996 (10.284, -48.792) -> (12.316, -48.792)
  arc A2267 (12.316, -48.8428) -> (12.316, -48.7412) centre (12.316, -48.792) ccw
  arc A2268 (10.284, -48.7412) -> (10.284, -48.8428) centre (10.284, -48.792) ccw
  line L997 (12.316, -48.792) -> (12.316, -49.808)
  arc A2269 (12.2652, -49.808) -> (12.3668, -49.808) centre (12.316, -49.808) ccw
  arc A2270 (12.3668, -48.792) -> (12.2652, -48.792) centre (12.316, -48.792) ccw
  line L998 (12.316, -49.808) -> (10.284, -49.808)
  arc A2271 (10.284, -49.7572) -> (10.284, -49.8588) centre (10.284, -49.808) ccw
  arc A2272 (12.316, -49.8588) -> (12.316, -49.7572) centre (12.316, -49.808) ccw
  line L999 (10.284, -49.808) -> (10.284, -48.792)
  arc A2273 (10.3348, -48.792) -> (10.2332, -48.792) centre (10.284, -48.792) ccw
  arc A2274 (10.2332, -49.808) -> (10.3348, -49.808) centre (10.284, -49.808) ccw
  arc A2275 (-18.3232, -40.12) -> (-18.3867, -40.12) centre (-18.355, -40.12) ccw
  line L1000 (2.584, -49.292) -> (4.616, -49.292)
  arc A2276 (4.616, -49.3428) -> (4.616, -49.2412) centre (4.616, -49.292) ccw
  arc A2277 (2.584, -49.2412) -> (2.584, -49.3428) centre (2.584, -49.292) ccw
  line L1001 (4.616, -49.292) -> (4.616, -50.308)
  arc A2278 (4.5652, -50.308) -> (4.6668, -50.308) centre (4.616, -50.308) ccw
  arc A2279 (4.6668, -49.292) -> (4.5652, -49.292) centre (4.616, -49.292) ccw
  line L1002 (4.616, -50.308) -> (2.584, -50.308)
  arc A2280 (2.584, -50.2572) -> (2.584, -50.3588) centre (2.584, -50.308) ccw
  arc A2281 (4.616, -50.3588) -> (4.616, -50.2572) centre (4.616, -50.308) ccw
  line L1003 (2.584, -50.308) -> (2.584, -49.292)
  arc A2282 (2.6348, -49.292) -> (2.5332, -49.292) centre (2.584, -49.292) ccw
  arc A2283 (2.5332, -50.308) -> (2.6348, -50.308) centre (2.584, -50.308) ccw
  arc A2284 (-18.3867, -53.28) -> (-18.3232, -53.28) centre (-18.355, -53.28) ccw
  line L1004 (6.608, -45.784) -> (6.608, -47.816)
  arc A2285 (6.5572, -47.816) -> (6.6588, -47.816) centre (6.608, -47.816) ccw
  arc A2286 (6.6588, -45.784) -> (6.5572, -45.784) centre (6.608, -45.784) ccw
  line L1005 (6.608, -47.816) -> (5.592, -47.816)
  arc A2287 (5.592, -47.7652) -> (5.592, -47.8668) centre (5.592, -47.816) ccw
  arc A2288 (6.608, -47.8668) -> (6.608, -47.7652) centre (6.608, -47.816) ccw
  line L1006 (5.592, -47.816) -> (5.592, -45.784)
  arc A2289 (5.6428, -45.784) -> (5.5412, -45.784) centre (5.592, -45.784) ccw
  arc A2290 (5.5412, -47.816) -> (5.6428, -47.816) centre (5.592, -47.816) ccw
  line L1007 (5.592, -45.784) -> (6.608, -45.784)
  arc A2291 (6.608, -45.8348) -> (6.608, -45.7332) centre (6.608, -45.784) ccw
  arc A2292 (5.592, -45.7332) -> (5.592, -45.8348) centre (5.592, -45.784) ccw
  arc A2293 (-4.22, -52.7148) -> (-4.22, -51.7252) centre (-4.22, -52.22) ccw
  line L1008 (10.116, -49.808) -> (8.084, -49.808)
  arc A2294 (8.084, -49.7572) -> (8.084, -49.8588) centre (8.084, -49.808) ccw
  arc A2295 (10.116, -49.8588) -> (10.116, -49.7572) centre (10.116, -49.808) ccw
  line L1009 (8.084, -49.808) -> (8.084, -48.792)
  arc A2296 (8.1348, -48.792) -> (8.0332, -48.792) centre (8.084, -48.792) ccw
  arc A2297 (8.0332, -49.808) -> (8.1348, -49.808) centre (8.084, -49.808) ccw
  line L1010 (8.084, -48.792) -> (10.116, -48.792)
  arc A2298 (10.116, -48.8428) -> (10.116, -48.7412) centre (10.116, -48.792) ccw
  arc A2299 (8.084, -48.7412) -> (8.084, -48.8428) centre (8.084, -48.792) ccw
  line L1011 (10.116, -48.792) -> (10.116, -49.808)
  arc A2300 (10.0652, -49.808) -> (10.1668, -49.808) centre (10.116, -49.808) ccw
  arc A2301 (10.1668, -48.792) -> (10.0652, -48.792) centre (10.116, -48.792) ccw
  arc A2302 (-4.22, -51.7252) -> (-4.22, -52.7148) centre (-4.22, -52.22) ccw
  line L1012 (2.616, -48.308) -> (0.584, -48.308)
  arc A2303 (0.584, -48.2572) -> (0.584, -48.3588) centre (0.584, -48.308) ccw
  arc A2304 (2.616, -48.3588) -> (2.616, -48.2572) centre (2.616, -48.308) ccw
  line L1013 (0.584, -48.308) -> (0.584, -47.292)
  arc A2305 (0.6348, -47.292) -> (0.5332, -47.292) centre (0.584, -47.292) ccw
  arc A2306 (0.5332, -48.308) -> (0.6348, -48.308) centre (0.584, -48.308) ccw
  line L1014 (0.584, -47.292) -> (2.616, -47.292)
  arc A2307 (2.616, -47.3428) -> (2.616, -47.2412) centre (2.616, -47.292) ccw
  arc A2308 (0.584, -47.2412) -> (0.584, -47.3428) centre (0.584, -47.292) ccw
  line L1015 (2.616, -47.292) -> (2.616, -48.308)
  arc A2309 (2.5652, -48.308) -> (2.6668, -48.308) centre (2.616, -48.308) ccw
  arc A2310 (2.6668, -47.292) -> (2.5652, -47.292) centre (2.616, -47.292) ccw
  arc A2311 (-4.22, -52.7148) -> (-4.22, -51.7252) centre (-4.22, -52.22) ccw
  line L1016 (6.892, -53.216) -> (6.892, -51.184)
  arc A2312 (6.9428, -51.184) -> (6.8412, -51.184) centre (6.892, -51.184) ccw
  arc A2313 (6.8412, -53.216) -> (6.9428, -53.216) centre (6.892, -53.216) ccw
  line L1017 (6.892, -51.184) -> (7.908, -51.184)
  arc A2314 (7.908, -51.2348) -> (7.908, -51.1332) centre (7.908, -51.184) ccw
  arc A2315 (6.892, -51.1332) -> (6.892, -51.2348) centre (6.892, -51.184) ccw
  line L1018 (7.908, -51.184) -> (7.908, -53.216)
  arc A2316 (7.8572, -53.216) -> (7.9588, -53.216) centre (7.908, -53.216) ccw
  arc A2317 (7.9588, -51.184) -> (7.8572, -51.184) centre (7.908, -51.184) ccw
  line L1019 (7.908, -53.216) -> (6.892, -53.216)
  arc A2318 (6.892, -53.1652) -> (6.892, -53.2668) centre (6.892, -53.216) ccw
  arc A2319 (7.908, -53.2668) -> (7.908, -53.1652) centre (7.908, -53.216) ccw
  arc A2320 (-4.22, -51.7252) -> (-4.22, -52.7148) centre (-4.22, -52.22) ccw
  line L1020 (2.997, -47.235) -> (0.203, -47.235)
  arc A2321 (0.203, -47.1842) -> (0.203, -47.2858) centre (0.203, -47.235) ccw
  arc A2322 (2.997, -47.2858) -> (2.997, -47.1842) centre (2.997, -47.235) ccw
  line L1021 (0.203, -47.235) -> (0.203, -45.965)
  arc A2323 (0.2538, -45.965) -> (0.1522, -45.965) centre (0.203, -45.965) ccw
  arc A2324 (0.1522, -47.235) -> (0.2538, -47.235) centre (0.203, -47.235) ccw
  line L1022 (0.203, -45.965) -> (2.997, -45.965)
  arc A2325 (2.997, -46.0158) -> (2.997, -45.9142) centre (2.997, -45.965) ccw
  arc A2326 (0.203, -45.9142) -> (0.203, -46.0158) centre (0.203, -45.965) ccw
  line L1023 (2.997, -45.965) -> (2.997, -47.235)
  arc A2327 (2.9462, -47.235) -> (3.0478, -47.235) centre (2.997, -47.235) ccw
  arc A2328 (3.0478, -45.965) -> (2.9462, -45.965) centre (2.997, -45.965) ccw
  line L1024 (-13.75, 1.2) -> (-16.25, 1.2)
  line L1025 (10.284, -49.792) -> (12.316, -49.792)
  arc A2329 (12.316, -49.8428) -> (12.316, -49.7412) centre (12.316, -49.792) ccw
  arc A2330 (10.284, -49.7412) -> (10.284, -49.8428) centre (10.284, -49.792) ccw
  line L1026 (12.316, -49.792) -> (12.316, -50.808)
  arc A2331 (12.2652, -50.808) -> (12.3668, -50.808) centre (12.316, -50.808) ccw
  arc A2332 (12.3668, -49.792) -> (12.2652, -49.792) centre (12.316, -49.792) ccw
  line L1027 (12.316, -50.808) -> (10.284, -50.808)
  arc A2333 (10.284, -50.7572) -> (10.284, -50.8588) centre (10.284, -50.808) ccw
  arc A2334 (12.316, -50.8588) -> (12.316, -50.7572) centre (12.316, -50.808) ccw
  line L1028 (10.284, -50.808) -> (10.284, -49.792)
  arc A2335 (10.3348, -49.792) -> (10.2332, -49.792) centre (10.284, -49.792) ccw
  arc A2336 (10.2332, -50.808) -> (10.3348, -50.808) centre (10.284, -50.808) ccw
  arc A2337 (-16.25, 1.2317) -> (-16.25, 1.1683) centre (-16.25, 1.2) ccw
  line L1029 (8.608, -45.784) -> (8.608, -47.816)
  arc A2338 (8.5572, -47.816) -> (8.6588, -47.816) centre (8.608, -47.816) ccw
  arc A2339 (8.6588, -45.784) -> (8.5572, -45.784) centre (8.608, -45.784) ccw
  line L1030 (8.608, -47.816) -> (7.592, -47.816)
  arc A2340 (7.592, -47.7652) -> (7.592, -47.8668) centre (7.592, -47.816) ccw
  arc A2341 (8.608, -47.8668) -> (8.608, -47.7652) centre (8.608, -47.816) ccw
  line L1031 (7.592, -47.816) -> (7.592, -45.784)
  arc A2342 (7.6428, -45.784) -> (7.5412, -45.784) centre (7.592, -45.784) ccw
  arc A2343 (7.5412, -47.816) -> (7.6428, -47.816) centre (7.592, -47.816) ccw
  line L1032 (7.592, -45.784) -> (8.608, -45.784)
  arc A2344 (8.608, -45.8348) -> (8.608, -45.7332) centre (8.608, -45.784) ccw
  arc A2345 (7.592, -45.7332) -> (7.592, -45.8348) centre (7.592, -45.784) ccw
  arc A2346 (-13.75, 1.1683) -> (-13.75, 1.2317) centre (-13.75, 1.2) ccw
  line L1033 (4.892, -53.216) -> (4.892, -51.184)
  arc A2347 (4.9428, -51.184) -> (4.8412, -51.184) centre (4.892, -51.184) ccw
  arc A2348 (4.8412, -53.216) -> (4.9428, -53.216) centre (4.892, -53.216) ccw
  line L1034 (4.892, -51.184) -> (5.908, -51.184)
  arc A2349 (5.908, -51.2348) -> (5.908, -51.1332) centre (5.908, -51.184) ccw
  arc A2350 (4.892, -51.1332) -> (4.892, -51.2348) centre (4.892, -51.184) ccw
  line L1035 (5.908, -51.184) -> (5.908, -53.216)
  arc A2351 (5.8572, -53.216) -> (5.9588, -53.216) centre (5.908, -53.216) ccw
  arc A2352 (5.9588, -51.184) -> (5.8572, -51.184) centre (5.908, -51.184) ccw
  line L1036 (5.908, -53.216) -> (4.892, -53.216)
  arc A2353 (4.892, -53.1652) -> (4.892, -53.2668) centre (4.892, -53.216) ccw
  arc A2354 (5.908, -53.2668) -> (5.908, -53.1652) centre (5.908, -53.216) ccw
  line L1037 (-16.25, 1.2) -> (-16.25, 3.2)
  line L1038 (9.903, -50.865) -> (12.697, -50.865)
  arc A2355 (12.697, -50.9158) -> (12.697, -50.8142) centre (12.697, -50.865) ccw
  arc A2356 (9.903, -50.8142) -> (9.903, -50.9158) centre (9.903, -50.865) ccw
  line L1039 (12.697, -50.865) -> (12.697, -52.135)
  arc A2357 (12.6462, -52.135) -> (12.7478, -52.135) centre (12.697, -52.135) ccw
  arc A2358 (12.7478, -50.865) -> (12.6462, -50.865) centre (12.697, -50.865) ccw
  line L1040 (12.697, -52.135) -> (9.903, -52.135)
  arc A2359 (9.903, -52.0842) -> (9.903, -52.1858) centre (9.903, -52.135) ccw
  arc A2360 (12.697, -52.1858) -> (12.697, -52.0842) centre (12.697, -52.135) ccw
  line L1041 (9.903, -52.135) -> (9.903, -50.865)
  arc A2361 (9.9538, -50.865) -> (9.8522, -50.865) centre (9.903, -50.865) ccw
  arc A2362 (9.8522, -52.135) -> (9.9538, -52.135) centre (9.903, -52.135) ccw
  arc A2363 (-16.2183, 3.2) -> (-16.2818, 3.2) centre (-16.2501, 3.2) ccw
  line L1042 (5.108, -45.784) -> (5.108, -47.816)
  arc A2364 (5.0572, -47.816) -> (5.1588, -47.816) centre (5.108, -47.816) ccw
  arc A2365 (5.1588, -45.784) -> (5.0572, -45.784) centre (5.108, -45.784) ccw
  line L1043 (5.108, -47.816) -> (4.092, -47.816)
  arc A2366 (4.092, -47.7652) -> (4.092, -47.8668) centre (4.092, -47.816) ccw
  arc A2367 (5.108, -47.8668) -> (5.108, -47.7652) centre (5.108, -47.816) ccw
  line L1044 (4.092, -47.816) -> (4.092, -45.784)
  arc A2368 (4.1428, -45.784) -> (4.0412, -45.784) centre (4.092, -45.784) ccw
  arc A2369 (4.0412, -47.816) -> (4.1428, -47.816) centre (4.092, -47.816) ccw
  line L1045 (4.092, -45.784) -> (5.108, -45.784)
  arc A2370 (5.108, -45.8348) -> (5.108, -45.7332) centre (5.108, -45.784) ccw
  arc A2371 (4.092, -45.7332) -> (4.092, -45.8348) centre (4.092, -45.784) ccw
  arc A2372 (-16.2818, 1.2) -> (-16.2183, 1.2) centre (-16.2501, 1.2) ccw
  line L1046 (10.608, -45.784) -> (10.608, -47.816)
  arc A2373 (10.5572, -47.816) -> (10.6588, -47.816) centre (10.608, -47.816) ccw
  arc A2374 (10.6588, -45.784) -> (10.5572, -45.784) centre (10.608, -45.784) ccw
  line L1047 (10.608, -47.816) -> (9.592, -47.816)
  arc A2375 (9.592, -47.7652) -> (9.592, -47.8668) centre (9.592, -47.816) ccw
  arc A2376 (10.608, -47.8668) -> (10.608, -47.7652) centre (10.608, -47.816) ccw
  line L1048 (9.592, -47.816) -> (9.592, -45.784)
  arc A2377 (9.6428, -45.784) -> (9.5412, -45.784) centre (9.592, -45.784) ccw
  arc A2378 (9.5412, -47.816) -> (9.6428, -47.816) centre (9.592, -47.816) ccw
  line L1049 (9.592, -45.784) -> (10.608, -45.784)
  arc A2379 (10.608, -45.8348) -> (10.608, -45.7332) centre (10.608, -45.784) ccw
  arc A2380 (9.592, -45.7332) -> (9.592, -45.8348) centre (9.592, -45.784) ccw
  line L1050 (-13.75, 3.2) -> (-13.75, 1.2)
  line L1051 (10.284, -52.092) -> (12.316, -52.092)
  arc A2381 (12.316, -52.1428) -> (12.316, -52.0412) centre (12.316, -52.092) ccw
  arc A2382 (10.284, -52.0412) -> (10.284, -52.1428) centre (10.284, -52.092) ccw
  line L1052 (12.316, -52.092) -> (12.316, -53.108)
  arc A2383 (12.2652, -53.108) -> (12.3668, -53.108) centre (12.316, -53.108) ccw
  arc A2384 (12.3668, -52.092) -> (12.2652, -52.092) centre (12.316, -52.092) ccw
  line L1053 (12.316, -53.108) -> (10.284, -53.108)
  arc A2385 (10.284, -53.0572) -> (10.284, -53.1588) centre (10.284, -53.108) ccw
  arc A2386 (12.316, -53.1588) -> (12.316, -53.0572) centre (12.316, -53.108) ccw
  line L1054 (10.284, -53.108) -> (10.284, -52.092)
  arc A2387 (10.3348, -52.092) -> (10.2332, -52.092) centre (10.284, -52.092) ccw
  arc A2388 (10.2332, -53.108) -> (10.3348, -53.108) centre (10.284, -53.108) ccw
  arc A2389 (-13.7818, 1.2) -> (-13.7183, 1.2) centre (-13.7501, 1.2) ccw
  line L1055 (7.603, -44.465) -> (10.397, -44.465)
  arc A2390 (10.397, -44.5158) -> (10.397, -44.4142) centre (10.397, -44.465) ccw
  arc A2391 (7.603, -44.4142) -> (7.603, -44.5158) centre (7.603, -44.465) ccw
  line L1056 (10.397, -44.465) -> (10.397, -45.735)
  arc A2392 (10.3462, -45.735) -> (10.4478, -45.735) centre (10.397, -45.735) ccw
  arc A2393 (10.4478, -44.465) -> (10.3462, -44.465) centre (10.397, -44.465) ccw
  line L1057 (10.397, -45.735) -> (7.603, -45.735)
  arc A2394 (7.603, -45.6842) -> (7.603, -45.7858) centre (7.603, -45.735) ccw
  arc A2395 (10.397, -45.7858) -> (10.397, -45.6842) centre (10.397, -45.735) ccw
  line L1058 (7.603, -45.735) -> (7.603, -44.465)
  arc A2396 (7.6538, -44.465) -> (7.5522, -44.465) centre (7.603, -44.465) ccw
  arc A2397 (7.5522, -45.735) -> (7.6538, -45.735) centre (7.603, -45.735) ccw
  arc A2398 (-13.7183, 3.2) -> (-13.7818, 3.2) centre (-13.7501, 3.2) ccw
  line L1059 (4.108, -45.784) -> (4.108, -47.816)
  arc A2399 (4.0572, -47.816) -> (4.1588, -47.816) centre (4.108, -47.816) ccw
  arc A2400 (4.1588, -45.784) -> (4.0572, -45.784) centre (4.108, -45.784) ccw
  line L1060 (4.108, -47.816) -> (3.092, -47.816)
  arc A2401 (3.092, -47.7652) -> (3.092, -47.8668) centre (3.092, -47.816) ccw
  arc A2402 (4.108, -47.8668) -> (4.108, -47.7652) centre (4.108, -47.816) ccw
  line L1061 (3.092, -47.816) -> (3.092, -45.784)
  arc A2403 (3.1428, -45.784) -> (3.0412, -45.784) centre (3.092, -45.784) ccw
  arc A2404 (3.0412, -47.816) -> (3.1428, -47.816) centre (3.092, -47.816) ccw
  line L1062 (3.092, -45.784) -> (4.108, -45.784)
  arc A2405 (4.108, -45.8348) -> (4.108, -45.7332) centre (4.108, -45.784) ccw
  arc A2406 (3.092, -45.7332) -> (3.092, -45.8348) centre (3.092, -45.784) ccw
  line L1063 (-16.25, 3.2) -> (-13.75, 3.2)
  line L1064 (2.592, -52.316) -> (2.592, -50.284)
  arc A2407 (2.6428, -50.284) -> (2.5412, -50.284) centre (2.592, -50.284) ccw
  arc A2408 (2.5412, -52.316) -> (2.6428, -52.316) centre (2.592, -52.316) ccw
  line L1065 (2.592, -50.284) -> (3.608, -50.284)
  arc A2409 (3.608, -50.3348) -> (3.608, -50.2332) centre (3.608, -50.284) ccw
  arc A2410 (2.592, -50.2332) -> (2.592, -50.3348) centre (2.592, -50.284) ccw
  line L1066 (3.608, -50.284) -> (3.608, -52.316)
  arc A2411 (3.5572, -52.316) -> (3.6588, -52.316) centre (3.608, -52.316) ccw
  arc A2412 (3.6588, -50.284) -> (3.5572, -50.284) centre (3.608, -50.284) ccw
  line L1067 (3.608, -52.316) -> (2.592, -52.316)
  arc A2413 (2.592, -52.2652) -> (2.592, -52.3668) centre (2.592, -52.316) ccw
  arc A2414 (3.608, -52.3668) -> (3.608, -52.2652) centre (3.608, -52.316) ccw
  arc A2415 (-13.75, 3.1683) -> (-13.75, 3.2317) centre (-13.75, 3.2) ccw
  line L1068 (3.665, -53.197) -> (3.665, -50.403)
  arc A2416 (3.7158, -50.403) -> (3.6142, -50.403) centre (3.665, -50.403) ccw
  arc A2417 (3.6142, -53.197) -> (3.7158, -53.197) centre (3.665, -53.197) ccw
  line L1069 (3.665, -50.403) -> (4.935, -50.403)
  arc A2418 (4.935, -50.4538) -> (4.935, -50.3522) centre (4.935, -50.403) ccw
  arc A2419 (3.665, -50.3522) -> (3.665, -50.4538) centre (3.665, -50.403) ccw
  line L1070 (4.935, -50.403) -> (4.935, -53.197)
  arc A2420 (4.8842, -53.197) -> (4.9858, -53.197) centre (4.935, -53.197) ccw
  arc A2421 (4.9858, -50.403) -> (4.8842, -50.403) centre (4.935, -50.403) ccw
  line L1071 (4.935, -53.197) -> (3.665, -53.197)
  arc A2422 (3.665, -53.1462) -> (3.665, -53.2478) centre (3.665, -53.197) ccw
  arc A2423 (4.935, -53.2478) -> (4.935, -53.1462) centre (4.935, -53.197) ccw
  arc A2424 (-16.25, 3.2317) -> (-16.25, 3.1683) centre (-16.25, 3.2) ccw
  line L1072 (-16.2108, -56.143) -> (-21.1892, -56.143)
  arc A2425 (-21.1892, -56.0922) -> (-21.1892, -56.1938) centre (-21.1892, -56.143) ccw
  arc A2426 (-16.2108, -56.1938) -> (-16.2108, -56.0922) centre (-16.2108, -56.143) ccw
  line L1073 (-21.1892, -56.143) -> (-21.1892, -53.857)
  arc A2427 (-21.1384, -53.857) -> (-21.24, -53.857) centre (-21.1892, -53.857) ccw
  arc A2428 (-21.24, -56.143) -> (-21.1384, -56.143) centre (-21.1892, -56.143) ccw
  line L1074 (-21.1892, -53.857) -> (-16.2108, -53.857)
  arc A2429 (-16.2108, -53.9078) -> (-16.2108, -53.8062) centre (-16.2108, -53.857) ccw
  arc A2430 (-21.1892, -53.8062) -> (-21.1892, -53.9078) centre (-21.1892, -53.857) ccw
  line L1075 (-16.2108, -53.857) -> (-16.2108, -56.143)
  arc A2431 (-16.2616, -56.143) -> (-16.16, -56.143) centre (-16.2108, -56.143) ccw
  arc A2432 (-16.16, -53.857) -> (-16.2616, -53.857) centre (-16.2108, -53.857) ccw
  arc A2433 (-15.9, 1.4793) -> (-15.9, 1.6207) centre (-15.9, 1.55) ccw
  line L1076 (41.707, 44.4108) -> (41.707, 49.3892)
  arc A2434 (41.7578, 49.3892) -> (41.6562, 49.3892) centre (41.707, 49.3892) ccw
  arc A2435 (41.6562, 44.4108) -> (41.7578, 44.4108) centre (41.707, 44.4108) ccw
  line L1077 (41.707, 49.3892) -> (43.993, 49.3892)
  arc A2436 (43.993, 49.3384) -> (43.993, 49.44) centre (43.993, 49.3892) ccw
  arc A2437 (41.707, 49.44) -> (41.707, 49.3384) centre (41.707, 49.3892) ccw
  line L1078 (43.993, 49.3892) -> (43.993, 44.4108)
  arc A2438 (43.9422, 44.4108) -> (44.0438, 44.4108) centre (43.993, 44.4108) ccw
  arc A2439 (44.0438, 49.3892) -> (43.9422, 49.3892) centre (43.993, 49.3892) ccw
  line L1079 (43.993, 44.4108) -> (41.707, 44.4108)
  arc A2440 (41.707, 44.4616) -> (41.707, 44.36) centre (41.707, 44.4108) ccw
  arc A2441 (43.993, 44.36) -> (43.993, 44.4616) centre (43.993, 44.4108) ccw
  arc A2442 (-15.9, 1.6207) -> (-15.9, 1.4793) centre (-15.9, 1.55) ccw
  line L1080 (57.485, 43.097) -> (57.485, 40.303)
  arc A2443 (57.4342, 40.303) -> (57.5358, 40.303) centre (57.485, 40.303) ccw
  arc A2444 (57.5358, 43.097) -> (57.4342, 43.097) centre (57.485, 43.097) ccw
  line L1081 (57.485, 40.303) -> (56.215, 40.303)
  arc A2445 (56.215, 40.3538) -> (56.215, 40.2522) centre (56.215, 40.303) ccw